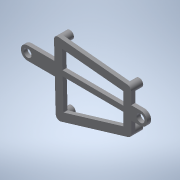
# Autodesk Inventor part: uno_holder
Saved by Autodesk Inventor 2020 (Build 240168000, 168)
## iProperties
Created: 2019-11-20
Part Number: uno_holder
Material: Generic
Document SubType Name: Modeling
Designer: psrob
Density: 1 g/cm^3
Appearance: Default
Author: psrob
Autodesk Inventor part; units mm, degrees
ref_plane "YZ Plane" through (0, 0, 0) normal (1, 0, 0) x (0, 1, 0)
ref_plane "XZ Plane" through (0, 0, 0) normal (0, 1, 0) x (-1, 0, 0)
ref_plane "XY Plane" through (0, 0, 0) normal (0, 0, 1) x (1, 0, 0)
sketch "Sketch1" plane through (0, 0, 0) normal (0, 0, 1) x (1, 0, 0)
  circle A0 centre (48.8243, -24.1116) radius 1.6 projected
  circle A1 centre (47.5543, 24.1484) radius 1.6 projected
  circle A2 centre (99.6243, 19.0684) radius 1.6 projected
  circle A3 centre (99.6243, -8.8716) radius 1.6 projected
  circle A4 centre (99.6243, -8.8716) radius 3
  circle A5 centre (47.5543, 24.1484) radius 3
  circle A6 centre (48.8243, -24.1116) radius 3
  circle A7 centre (99.6243, 19.0684) radius 3
  point P0 (0, 0)
  dimension "d0" = 6
  dimension "d1" = 6
  dimension "d2" = 6
  dimension "d3" = 6
  constraints: 4 centre point, 4 coincident
  measures "d0" diameter of A4
  measures "d1" diameter of A5
  measures "d2" diameter of A6
  measures "d3" diameter of A7
extrude "Extrusion1" add sketch "Sketch1" along normal blind 6
sketch "Sketch2" plane through (99.6243, -8.8716, 6) normal (0, 0, 1) x (1, 0, 0)
  circle A0 centre (0, 0) radius 3 projected
  circle A1 centre (0, 0) radius 1.6 projected
  circle A2 centre (0, 27.94) radius 3 projected
  circle A3 centre (0, 27.94) radius 3 projected
  circle A4 centre (0, 27.94) radius 1.6 projected
  circle A5 centre (-52.07, 33.02) radius 3 projected
  circle A6 centre (-52.07, 33.02) radius 1.6 projected
  circle A7 centre (-50.8, -15.24) radius 3 projected
  circle A8 centre (-50.8, -15.24) radius 1.6 projected
  circle A9 centre (0, 0) radius 1.6 projected
  circle A10 centre (-50.8, -15.24) radius 1.6 projected
  line L0 (0, 0) -> (-50.8, -15.24)
  circle A11 centre (-52.07, 33.02) radius 3 projected
  line L1 (-50.8, -15.24) -> (-52.07, 33.02)
  circle A12 centre (0, 27.94) radius 1.6 projected
  line L2 (-52.07, 33.02) -> (0, 27.94)
  line L3 (0, 27.94) -> (0, 0)
  line L4 (0, 0) -> (-50.8, -15.24) construction
  line L5 (0.862, -2.8735) -> (-49.938, -18.1135)
  line L6 (-51.662, -12.3665) -> (-0.862, 2.8735)
  arc A13 (0.862, -2.8735) -> (-0.862, 2.8735) centre (0, 0) ccw
  arc A14 (-51.662, -12.3665) -> (-49.938, -18.1135) centre (-50.8, -15.24) ccw
  circle A15 centre (-52.07, 33.02) radius 1.6 projected
  line L7 (-50.8, -15.24) -> (-52.07, 33.02) construction
  line L8 (-47.801, -15.1611) -> (-49.071, 33.0989)
  line L9 (-55.069, 32.9411) -> (-53.799, -15.3189)
  arc A16 (-53.799, -15.3189) -> (-47.801, -15.1611) centre (-50.8, -15.24) ccw
  arc A17 (-49.071, 33.0989) -> (-55.069, 32.9411) centre (-52.07, 33.02) ccw
  line L10 (0, 27.94) -> (-52.07, 33.02) construction
  line L11 (0.2913, 30.9258) -> (-51.7787, 36.0058)
  line L12 (-52.3613, 30.0342) -> (-0.2913, 24.9542)
  arc A18 (-0.2913, 24.9542) -> (0.2913, 30.9258) centre (0, 27.94) ccw
  arc A19 (-51.7787, 36.0058) -> (-52.3613, 30.0342) centre (-52.07, 33.02) ccw
  line L13 (0, 0) -> (0, 27.94) construction
  line L14 (3, 0) -> (3, 27.94)
  line L15 (-3, 27.94) -> (-3, 0)
  arc A20 (-3, 0) -> (3, 0) centre (0, 0) ccw
  arc A21 (3, 27.94) -> (-3, 27.94) centre (0, 27.94) ccw
  point P0 (-99.6243, 8.8716)
  point P1 (-25.4, -7.62)
  point P2 (-51.435, 8.89)
  point P3 (-26.035, 30.48)
  point P4 (0, 13.97)
  point P5 (0.862, -2.8735)
  point P6 (3, 0)
  point P7 (3, 27.94)
  point P8 (0.2913, 30.9258)
  point P9 (-51.7787, 36.0058)
  point P10 (-47.9042, -11.2392)
  point P11 (-48.9817, 29.7045)
  point P12 (-3, 25.2184)
  point P13 (-3, 2.2321)
  dimension "d6" = 3
  constraints: 40 end point, 16 point on circle, 16 tangent, 8 centre point, 8 midpoint, 6 equal length, 2 concentric, 1 vertical
  measures "d6" radius of A13
extrude "Extrusion2" add sketch "Sketch2" along normal blind 3 contours A0 L3 A1 L0 | L6 L15 L12 A2 L3 A0 | A0 L15 L6 | A0 L0 L8 L6 L15 | L3 A2 L14 A0 | A0 L0 A1 L3 | A0 L5 A7 L8 L0 | L3 A4 L2 A2 | A2 L2 A4 L3 | L3 L0 A1 | A1 L0 L3 | L8 L0 A7 L1 L6 | L6 L1 L12 L8 | L15 A2 L12 | L12 L8 L2 A2 L15 | L8 A7 L0 | L3 L2 A4 | A4 L2 L3 | L6 A7 L9 A5 L12 L1 | L1 A7 L6 | L12 L1 A5 L2 L8 | A7 L1 A8 L0 | L0 A8 L1 A7 | A2 L2 L8 A5 L11 | L12 A5 L1 | L2 A5 L8 | L0 L1 A8 | A8 L1 L0 | A5 L2 A6 L1 | L1 A6 L2 A5 | L1 L2 A6 | A6 L2 L1
sketch "Sketch3" plane through (99.6243, -8.8716, 9) normal (0, 0, 1) x (1, 0, 0)
  arc A0 (3, 27.94) -> (0.2913, 30.9258) centre (0, 27.94) ccw projected
  line L0 (0.2913, 30.9258) -> (-51.7787, 36.0058) projected
  arc A1 (-51.7787, 36.0058) -> (-55.069, 32.9411) centre (-52.07, 33.02) ccw projected
  line L1 (-55.069, 32.9411) -> (-53.799, -15.3189) projected
  arc A2 (-53.799, -15.3189) -> (-49.938, -18.1135) centre (-50.8, -15.24) ccw projected
  line L2 (-49.938, -18.1135) -> (0.862, -2.8735) projected
  arc A3 (0.862, -2.8735) -> (3, 0) centre (0, 0) ccw projected
  line L3 (3, 0) -> (3, 27.94) projected
  line L4 (-3, 25.2184) -> (-3, 2.2321) projected
  line L5 (-3, 2.2321) -> (-47.9042, -11.2392) projected
  line L6 (-47.9042, -11.2392) -> (-48.9817, 29.7045) projected
  line L7 (-48.9817, 29.7045) -> (-3, 25.2184) projected
  circle A4 centre (0, 27.94) radius 1.6 projected
  line L8 (0, 0) -> (0, 27.94)
  line L9 (0, 27.94) -> (0, 13.97)
  line L10 (0, 13.97) -> (10, 13.97)
  line L11 (0, 13.97) -> (-75, 13.97)
  line L12 (10, 13.97) -> (-75, 13.97) construction
  line L13 (10, 18.97) -> (-75, 18.97)
  line L14 (-75, 8.97) -> (10, 8.97)
  arc A5 (10, 8.97) -> (10, 18.97) centre (10, 13.97) ccw
  arc A6 (-75, 18.97) -> (-75, 8.97) centre (-75, 13.97) ccw
  circle A7 centre (10, 13.97) radius 3
  circle A8 centre (-75, 13.97) radius 3
  line L15 (-3, 25.2184) -> (-3, 2.2321) projected
  line L16 (-3, 13.7253) -> (-48.5676, 13.97) construction
  line L17 (-2.9893, 15.7252) -> (-48.5569, 15.97)
  line L18 (-48.5784, 11.97) -> (-3.0107, 11.7253)
  arc A9 (-3.0107, 11.7253) -> (-2.9893, 15.7252) centre (-3, 13.7253) ccw
  arc A10 (-48.5569, 15.97) -> (-48.5784, 11.97) centre (-48.5676, 13.97) ccw
  point P0 (-99.6243, 8.8716)
  point P1 (-32.5, 13.97)
  point P2 (-25.7838, 13.8476)
  point P3 (-54.7013, 18.97)
  point P4 (-54.4381, 8.97)
  point P5 (3, 8.97)
  point P6 (3, 18.97)
  dimension "d9" = 10
  dimension "d10" = 75
  dimension "d11" = 10
  dimension "d12" = 6
  dimension "d13" = 6
  dimension "d14" = 4
  constraints: 24 end point, 8 point on circle, 8 tangent, 6 centre point, 4 midpoint, 2 coincident, 2 horizontal, 2 parallel, 2 point on line, 1 perpendicular, 1 vertical
  measures "d9" distance of L9.end L10.end
  measures "d10" distance of L9.end L11.end
  measures "d11" diameter of A6
  measures "d12" diameter of A7
  measures "d13" diameter of A8
  measures "d14" diameter of A10
extrude "Extrusion3" add sketch "Sketch3" against normal up to surface (3 mm away) contours L13 A5 L14 L3 | L1 L14 A6 L13 | A9 L4 L11 | L11 L4 L17 A9 | L4 L11 L6 A10 L17 | L4 A9 L18 L6 L11 | L6 L11 A10 | L11 L6 L18 A10
body "Solid1"
